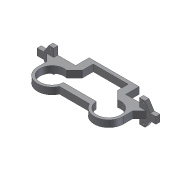
# Autodesk Inventor part: Suporte - Baterias
Saved by Autodesk Inventor 2011 (Build 150239000, 239)
## iProperties
Created: 2011-04-09
Part Number: Suporte - Baterias
Document SubType Name: Modeling
Designer: Milton
Density: 1 g/cm^3
Author: Milton
Autodesk Inventor part; units mm, degrees
ref_plane "YZ Plane" through (0, 0, 0) normal (1, 0, 0) x (0, 1, 0)
ref_plane "XZ Plane" through (0, 0, 0) normal (0, 1, 0) x (-1, 0, 0)
ref_plane "XY Plane" through (0, 0, 0) normal (0, 0, 1) x (1, 0, 0)
sketch "Sketch1" plane through (0, 0, 0) normal (0, 0, 1) x (1, 0, 0)
  circle A0 centre (54.75, -22.5111) radius 17.75
  circle A1 centre (-29.25, -22.5111) radius 17.75
  arc A2 (33.2627, -23.2512) -> (47.5068, -2.2679) centre (54.75, -22.5111) ccw
  arc A3 (-22.0068, -2.2679) -> (-7.7627, -23.2512) centre (-29.25, -22.5111) ccw
  line L0 (-24.25, 7.4889) -> (-75.25, 7.4889)
  line L1 (49.75, 27.4889) -> (49.75, 7.4889)
  line L2 (-24.25, 27.4889) -> (-24.25, 7.4889)
  line L3 (-75.25, 7.4908) -> (-75.25, 1.4889)
  line L4 (100.75, 1.4889) -> (100.75, 7.4889)
  line L5 (49.75, 7.4889) -> (100.75, 7.4889)
  line L6 (49.75, 27.4889) -> (-24.25, 27.4889)
  line L7 (38.75, 22.4889) -> (-13.25, 22.4889)
  line L8 (38.75, 22.4889) -> (38.75, 6.4889)
  line L9 (-13.25, 22.4889) -> (-13.25, 6.4889)
  line L10 (-13.25, 6.4889) -> (22.1216, 6.4889) construction
  line L11 (-11.5154, -23.2512) -> (37.0154, -23.2512)
  line L12 (38.75, 6.4889) -> (77.4628, 6.4889) construction
  line L13 (-13.25, 6.4889) -> (-25.0131, -5.2742)
  line L14 (-13.25, 6.4889) -> (21.7518, 6.4889) construction
  line L15 (38.75, 6.4889) -> (50.5131, -5.2742)
  line L16 (38.75, 6.4889) -> (73.7518, 6.4889) construction
  line L17 (-9.6067, -31.2512) -> (35.1067, -31.2512)
  line L18 (-75.25, 1.4889) -> (-60.75, 1.4889)
  line L19 (-50.75, -22.5111) -> (-50.75, -8.5111)
  line L20 (76.25, -22.5111) -> (76.25, -8.5111)
  line L21 (86.25, 1.4889) -> (100.75, 1.4889)
  line L22 (-60.75, 1.4889) -> (-50.75, -8.5111)
  line L23 (86.25, 1.4889) -> (76.25, -8.5111)
  point P0 (0, 0)
  point P1 (-50.75, 1.4889)
  point P2 (76.25, 1.4889)
  dimension "d6" = 35.5
  dimension "d7" = 35.5
  dimension "d14" = 43
  dimension "d15" = 43
  dimension "d40" = 5
  dimension "d41" = 11
  dimension "d42" = 11
  dimension "d43" = 52
  dimension "d44" = 16
  dimension "d45" = 16
  dimension "d47" = 16
  dimension "d49" = 16
  dimension "d52" = 30
  dimension "d53" = 30
  dimension "d55" = 20
  dimension "d56" = 20
  dimension "d57" = 135
  dimension "d59" = 45
  dimension "d60" = 46
  dimension "d61" = 46
  dimension "d62" = 8
  dimension "d82" = 6
  dimension "d83" = 6
  dimension "d87" = 10
  dimension "d88" = 10
  dimension "d89" = 10
  dimension "d90" = 10
  constraints: 48 end point, 12 point on circle, 9 point on line, 8 parallel, 4 centre point, 4 horizontal, 4 perpendicular, 2 coincident, 2 tangent
  measures "d6" diameter of A0
  measures "d7" diameter of A1
  measures "d14" diameter of A2
  measures "d15" diameter of A3
  measures "d40" distance between parallel lines of L6 L7
  measures "d41" distance between parallel lines of L8 L1
  measures "d42" distance between parallel lines of L2 L9
  measures "d43" distance of L7.start L7.end
  measures "d44" distance from line of A1.centre L9
  measures "d45" distance from line of L8 A0.centre
  measures "d47" distance of L7.end L9.end
  measures "d49" distance of L7.start L8.end
  measures "d52" distance from line of L5 A2.centre
  measures "d53" distance from line of L0 A1.centre
  measures "d55" distance between parallel lines of L0 L6
  measures "d56" distance of L1.start L1.end
  measures "d57" angle of L13 L14
  measures "d59" angle of L15 L16
  measures "d60" distance from line of L3 A1.centre
  measures "d61" distance from line of L4 A0.centre
  measures "d62" distance between parallel lines of L17 L11
  measures "d82" distance between parallel lines of L18 L0
  measures "d83" distance between parallel lines of L21 L5
  measures "d87" distance of L18.end point (-50.75, 1.489)
  measures "d88" distance of L19.end point (-50.75, 1.489)
  measures "d89" distance of L21.start point (76.25, 1.489)
  measures "d90" distance of L20.end point (76.25, 1.489)
extrude "Extrusion1" add sketch "Sketch1" along normal blind 10 contours A0 L15 A2 L11 | L15 L8 L7 L9 L13 A3 L19 L22 L18 L3 L0 L2 L6 L1 L5 L4 L21 L23 L20 A2 | A2 L17 A3 L11 | A3 L13 A1 L11
sketch "Sketch3" plane through (-75.25, 7.4889, 0) normal (0, 1, 0) x (1, 0, 0)
  line L0 (51, 0) -> (0, 0) projected
  circle A0 centre (19.367, -18.7742) radius 1.5
  circle A1 centre (19.367, 8.774) radius 1.5
  line L1 (17.2888, -22) -> (9.4959, -10)
  line L2 (9.4958, 0) -> (17.2888, 12)
  line L3 (17.2888, 12) -> (24.5, 12)
  line L4 (24.5, 12) -> (24.5, 0)
  circle A2 centre (157.6308, -18.7741) radius 1.5
  circle A3 centre (157.6308, 8.7741) radius 1.5
  line L5 (159.7093, -22) -> (167.5022, -10)
  line L6 (176, -10) -> (130, -10) projected
  line L7 (159.7093, -22) -> (174.0176, -22) construction
  line L8 (151.5, -10) -> (151.5, -22)
  line L9 (151.5, -22) -> (159.7093, -22)
  line L10 (151.5, 12) -> (159.7093, 11.9999)
  line L11 (159.7093, 11.9999) -> (167.502, 0)
  line L12 (130, 0) -> (176, 0) projected
  line L13 (24.5, 0) -> (9.4958, 0)
  line L14 (151.5, 12) -> (151.5, 0)
  line L15 (151.5, 0) -> (167.502, 0)
  line L16 (151.5, -10) -> (167.5022, -10)
  line L17 (0, -10) -> (51, -10) projected
  line L18 (24.5, -10) -> (24.5, -22)
  line L19 (24.5, 0) -> (24.5, -10) projected
  line L20 (17.2888, -22) -> (24.5, -22)
  line L21 (9.4959, -10) -> (24.5, -10)
  line L22 (151.5, 0) -> (151.5, -10) projected
  point P0 (75.25, 0)
  dimension "d63" = 3
  dimension "d64" = 3
  dimension "d69" = 12
  dimension "d70" = 3
  dimension "d71" = 3
  dimension "d72" = 57
  dimension "d74" = 12
  dimension "d77" = 123
  constraints: 34 end point, 6 point on line, 4 centre point, 4 collinear, 4 perpendicular, 1 equal length, 1 horizontal
  measures "d63" diameter of A0
  measures "d64" diameter of A1
  measures "d69" distance of L3.end L4.end
  measures "d70" diameter of A2
  measures "d71" diameter of A3
  measures "d72" angle of L7 L5
  measures "d74" distance of L8.start L8.end
  measures "d77" angle of L10 L11
extrude "Extrusion3" add sketch "Sketch3" against normal blind 6
equation "\"d88\" = d87"
equation "\"d89\" = d87"
equation "\"d90\" = d89"
body "Solid1"
